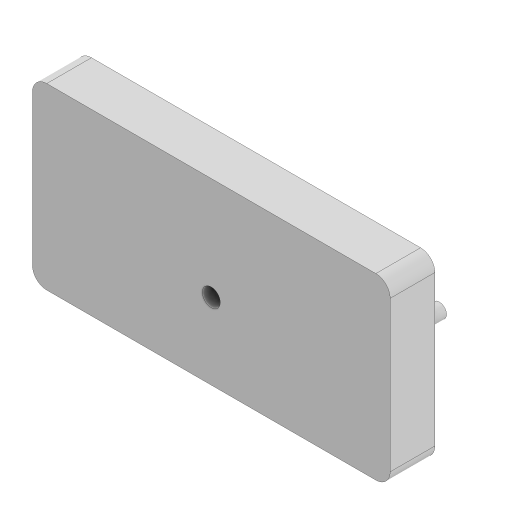
# Autodesk Inventor part: CAJA REDUCTORA
Saved by Autodesk Inventor 2024 (Build 280153000, 153)
## iProperties
Created: 2024-08-15
Part Number: CAJA REDUCTORA
Material: Generic
Document SubType Name: Modeling
Designer: Jhuliams
Density: 1 g/cm^3
Appearance: Default
Author: Jhuliams
Autodesk Inventor part; units mm, degrees
ref_plane "YZ Plane" through (0, 0, 0) normal (1, 0, 0) x (0, 1, 0)
ref_plane "XZ Plane" through (0, 0, 0) normal (0, 1, 0) x (-1, 0, 0)
ref_plane "XY Plane" through (0, 0, 0) normal (0, 0, 1) x (1, 0, 0)
sketch "Sketch1" plane through (0, 0, 0) normal (0, 0, 1) x (1, 0, 0)
  line L0 (-100, 50) -> (100, 50)
  line L1 (100, 50) -> (100, -50)
  line L2 (100, -50) -> (-100, -50)
  line L3 (-100, -50) -> (-100, 50)
  line L4 (-100, 50) -> (100, -50) construction
  line L5 (100, 50) -> (-100, -50) construction
  point P0 (0, 0)
  dimension "d0" = 200
  dimension "d1" = 100
  constraints: 12 end point, 2 midpoint, 2 parallel, 1 horizontal, 1 perpendicular
  measures "d0" distance of L1.end L2.end
  measures "d1" distance of L0.end L1.end
extrude "Extrusion1" add sketch "Sketch1" along normal mid plane 25
fillet "Fillet1" radius 8 4 edges at (100, 50, 0) (-100, 50, 0) (100, -50, 0) (-100, -50, 0)
sketch "Sketch2" plane through (0, 0, -12.5) normal (0, 0, -1) x (-1, 0, 0)
  line L0 (-77.5, 10) -> (77.5, 10)
  line L1 (77.5, 10) -> (77.5, -10)
  line L2 (77.5, -10) -> (-77.5, -10)
  line L3 (-77.5, -10) -> (-77.5, 10)
  line L4 (-77.5, 10) -> (77.5, -10) construction
  line L5 (77.5, 10) -> (-77.5, -10) construction
  circle A0 centre (-77.5, 0) radius 4
  circle A1 centre (77.5, 0) radius 4
  point P0 (0, 0)
  dimension "d5" = 155
  dimension "d6" = 20
  dimension "d7" = 8
  dimension "d8" = 8
  constraints: 12 end point, 4 midpoint, 2 centre point, 2 parallel, 1 horizontal, 1 perpendicular
  measures "d5" distance of L1.end L2.end
  measures "d6" distance of L0.end L1.end
  measures "d7" diameter of A0
  measures "d8" diameter of A1
extrude "Extrusion2" add sketch "Sketch2" along normal blind 25 contours A0 L3 | L3 A0 | A1 L1 | L1 A1
sketch "Sketch3" plane through (0, 0, -12.5) normal (0, 0, -1) x (-1, 0, 0)
  line L0 (-92, -50) -> (92, -50) projected
  line L1 (0, -50) -> (0, -7.5)
  circle A0 centre (0, -7.5) radius 5
  point P0 (0, 0)
  dimension "d11" = 42.5
  dimension "d12" = 10
  constraints: 2 end point, 1 centre point, 1 coincident, 1 midpoint, 1 vertical
  measures "d11" distance of L1.start L1.end
  measures "d12" diameter of A0
extrude "Extrusion3" cut sketch "Sketch3" against normal blind 25
body "Solid1"
